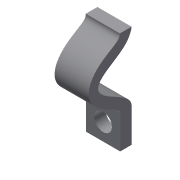
# Autodesk Inventor part: 20_Cube_Insert_Z-Focus_Sampleclamp
Saved by Autodesk Inventor 2019.4 (Build 234330000, 330)
## iProperties
Created: 2021-02-06
Part Number: 20_Cube_Insert_Z-Focus_Sampleclamp
Material: Generic
Document SubType Name: Modeling
Designer: diederichbenedict
Density: 1 g/cm^3
Appearance: Default
Author: diederichbenedict
Autodesk Inventor part; units mm, degrees
ref_plane "YZ Plane" through (0, 0, 0) normal (1, 0, 0) x (0, 1, 0)
ref_plane "XZ Plane" through (0, 0, 0) normal (0, 1, 0) x (-1, 0, 0)
ref_plane "XY Plane" through (0, 0, 0) normal (0, 0, 1) x (1, 0, 0)
sketch "Sketch1" plane through (0, 0, 0) normal (1, 0, 0) x (0, 1, 0)
  line L0 (74.4881, 0) -> (80.4881, 0)
  line L1 (80.4881, 0) -> (80.4881, 2)
  line L2 (80.4881, 2) -> (74.4881, 2)
  line L3 (74.4881, 2) -> (74.4881, 0)
  line L4 (80.4881, 0) -> (82.3869, 0) construction
  line L5 (82.3869, 0) -> (84.266, 7.0131) construction
  line L6 (84.266, 7.0131) -> (87.8067, 7.0131) construction
  line L7 (87.8067, 7.0131) -> (89.6859, 0) construction
  line L8 (89.6859, 0) -> (92.5076, 0) construction
  line L9 (92.5076, 0) -> (92.4881, 0) construction
  spline S0 degree 4 poles (80.4881, 0) (82.3869, 0) (84.266, 7.0131) (87.8067, 7.0131) (89.6859, 0) (92.5076, 0) (92.4881, 0) knots 1 1 1 1 1 2 3 4 4 4 4 4
  line L10 (80.4881, 2) -> (81.1356, 1.6906) construction
  line L11 (81.1356, 1.6906) -> (82.7335, 8.6116) construction
  line L12 (82.7335, 8.6116) -> (89.449, 8.6116) construction
  line L13 (89.449, 8.6116) -> (91.2062, 2.0534) construction
  line L14 (91.2062, 2.0534) -> (92.0512, 2.0534) construction
  line L15 (92.0512, 2.0534) -> (92.4881, 2.0534) construction
  spline S1 degree 4 poles (80.4881, 2) (81.1356, 1.6906) (82.7335, 8.6116) (89.449, 8.6116) (91.2062, 2.0534) (92.0512, 2.0534) (92.4881, 2.0534) knots 1 1 1 1 1 2 3 4 4 4 4 4
  line L16 (92.4881, 2.0534) -> (92.4881, 0)
  point P0 (0, 0)
  dimension "d0" = 6
  dimension "d1" = 2
  dimension "d2" = 0
  dimension "d8" = 12
  dimension "d9" = 0
  dimension "d10" = 2
  dimension "d11" = 2
  dimension "d12" = 15
  dimension "d13" = 165
  constraints: 10 end point, 6 parallel, 5 horizontal, 1 collinear, 1 perpendicular, 1 point on line, 9 other
  measures "d0" distance of L1.end L2.end
  measures "d1" distance of L1.end L0.end
  measures "d2" distance from line of L0 point (0, 0)
  measures "d8" distance between parallel lines of L16 L1
  measures "d9" distance from line of L9.end L0
  measures "d10" angle of L5 L11
  measures "d11" distance between parallel lines of L13 L7
  measures "d12" angle of L5 L1
  measures "d13" angle of L7 L1
extrude "Extrusion1" add sketch "Sketch1" along normal blind 6
sketch "Sketch2" plane through (0, 74.4881, 2) normal (0, 0, 1) x (1, 0, 0)
  line L0 (0, 6) -> (0, 0) projected
  line L1 (0, 0) -> (6, 0) projected
  line L2 (6, 6) -> (6, 0) projected
  line L3 (0, 6) -> (6, 6) projected
  circle A0 centre (3, 3) radius 1.55
  point P0 (0, -74.4881)
  dimension "d5" = 3.1
  constraints: 1 centre point
  measures "d5" diameter of A0
extrude "Extrusion2" cut sketch "Sketch2" against normal blind 6 contours A0
body "Solid1"
